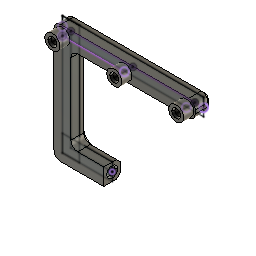
ThymioPipeRight (Autodesk Fusion 360 design; units mm, degrees)
part number: 2026-07-25-12-46-37-423
Autodesk Fusion 360 part; units mm, degrees
sketch "Sketch1" plane through (0, 0, 0) normal (0, 1, 0) x (1, 0, 0)
  line L0 (0, 0) -> (-20, 0)
  line L1 (-20, 0) -> (-20, -49)
  line L2 (-20, -49) -> (10, -49)
  line L3 (10, -49) -> (40, -49)
  line L4 (0, -4.1) -> (-24.1, -4.1)
  line L5 (-24.1, -4.1) -> (-24.1, 4.1)
  line L6 (-24.1, 4.1) -> (0, 4.1)
  line L7 (0, 4.1) -> (0, -4.1)
  line L8 (-24.1, 4.1) -> (-15.9, 4.1)
  line L9 (-15.9, 4.1) -> (-15.9, -53.4)
  line L10 (-15.9, -53.4) -> (-24.1, -53.4)
  line L11 (-24.1, -53.4) -> (-24.1, 4.1)
  line L12 (-24.1, -53.4) -> (44.3, -53.4)
  line L13 (44.3, -53.4) -> (44.3, -45.2)
  line L14 (44.3, -45.2) -> (-24.1, -45.2)
  line L15 (-24.1, -45.2) -> (-24.1, -53.4)
  dimension "d10" = 20
  dimension "d11" = 49
  dimension "d12" = 30
  dimension "d13" = 30
  dimension "d14" = 8.2
  dimension "d15" = 24.1
  dimension "d16" = 57.5
  dimension "d18" = 68.4
  dimension "d19" = 8.2
  dimension "d20" = 8.2
  constraint coincident L0.start origin
  constraint horizontal L0
  constraint vertical L1
  constraint horizontal L3
  constraint horizontal L2
  constraint horizontal L4
  constraint vertical L5
  constraint horizontal L6
  constraint vertical L7
  constraint midpoint L0.start L7
  constraint horizontal L8
  constraint vertical L9
  constraint horizontal L10
  constraint vertical L11
  constraint horizontal L12
  constraint vertical L13
  constraint horizontal L14
  constraint vertical L15
  measures "d10" distance of L0.start L0.end
  measures "d11" distance of L0.end L1.end
  measures "d12" distance of L1.end L2.end
  measures "d13" distance of L2.end L3.end
  measures "d14" distance of L4.start L6.end
  measures "d15" distance of L5 L7
  measures "d16" distance of L6 L10
  measures "d18" distance of L13 L15
  measures "d19" distance of L12 L14
  measures "d20" distance of L9 L11
extrude "Extrude1" add sketch "Sketch1" along normal mid plane 8.2
sketch "Sketch2" plane through (0, -4.1, 0) normal (0, -1, 0) x (1, 0, 0)
  line L0 (-24.1, 53.4) -> (-24.1, -4.1)
  line L1 (-24.1, -4.1) -> (0, -4.1)
  line L2 (0, -4.1) -> (0, 4.1)
  line L3 (0, 4.1) -> (-15.9, 4.1)
  line L4 (-15.9, 4.1) -> (-15.9, 45.2)
  line L5 (-15.9, 45.2) -> (44.3, 45.2)
  line L6 (44.3, 45.2) -> (44.3, 53.4)
  line L7 (44.3, 53.4) -> (-24.1, 53.4)
  line L8 (-20, 49) -> (10, 49)
  line L9 (10, 49) -> (40, 49)
  circle A0 centre (-20, 49) radius 3.625
  circle A1 centre (10, 49) radius 3.625
  circle A2 centre (40, 49) radius 3.625
  point P0 (10, 49)
  point P1 (40, 49)
  dimension "d23" = 7.25
  dimension "d24" = 7.25
  dimension "d25" = 7.25
  constraint coincident L8.start A0.centre
  constraint coincident P0 L8.end
  constraint coincident P1 L9.end
  measures "d23" diameter of A0
  measures "d24" diameter of A1
  measures "d25" diameter of A2
ref_plane "WorkPlane1" through (0, 0, 49) normal (0, 0, 1) x (1, 0, 0)
sketch "Sketch3" plane through (0, 0, 49) normal (0, 0, 1) x (1, 0, 0)
  line L0 (40, 0) -> (40, -9)
  line L1 (10, 0) -> (10, -9)
  line L2 (-20, 0) -> (-20, -9)
  line L3 (-24.1, 0) -> (44.3, 0)
  line L4 (-20, -4.1) -> (10, -4.1)
  point P0 (-20, -4.1)
  point P1 (10, -4.1)
  point P2 (40, -4.1)
  point P3 (-20, 0)
  point P4 (10, 0)
  point P5 (40, 0)
  dimension "d31" = 9
  dimension "d32" = 9
  dimension "d33" = 9
  constraint vertical L0
  constraint vertical L1
  constraint vertical L2
  constraint coincident L2 P0
  constraint coincident P5 L3
  constraint coincident P3 L2.start
  constraint coincident L1.start P4
  constraint coincident P5 L0.start
  measures "d31" distance of P5 L0.end
  measures "d32" distance of L1.end L1.start
  measures "d33" distance of L2.end P3
extrude "Extrude2" add sketch "Sketch2" along normal blind 4.9 contours L8 L9 A1 | L8 L9 A1 | A0 | A2
pipe "Pipe1" cut diameter 4.2 path "Sketch1" along L0 L1 L2 L3
pipe "Pipe2" cut diameter 3.25 path "Sketch3" along L2
pipe "Pipe3" cut diameter 3.25 path "Sketch3" along L1
pipe "Pipe4" cut diameter 3.25 path "Sketch3" along L0
fillet "Fillet1" offset 0.5 second offset 1 3 edges at (8.485, -9, 49.5876) (-21.515, -9, 49.5876) (38.485, -9, 49.5876) measured on face at (12.9388, -9, 49.2608) measured on face at (-17.0567, -9, 48.7794) measured on face at (42.9433, -9, 49.2206)
fillet "Fillet1" offset 0.5 second offset 1 1 edges at (0, 1.9579, -0.7594) measured on face at (0, 3.4314, 0.0523)
fillet "Fillet2" radius 3.25 6 edges at (-15.9, 0, 45.2) (44.3, 0, 45.2) (44.3, 0, 53.4) (-24.1, 0, 53.4) (-24.1, 0, -4.1) (-15.9, 0, 4.1)
sketch "Sketch4" plane through (0, 4.1, 0) normal (0, 1, 0) x (1, 0, 0)
  line L0 (-12.0349, 3.5252) -> (-22.5468, 3.5252) construction
  line L1 (-22.5468, 3.5252) -> (-22.5468, -4.1335) construction
  line L2 (-22.5468, -4.1335) -> (-12.0349, -4.1335) construction
  line L3 (-12.0349, -4.1335) -> (-12.0349, 3.5252) construction
  arc A0 (-21.1, 4.1) -> (-24.1, 1.1) centre (-21.1, 1.1) ccw
  line L4 (-24.1, 1.1) -> (-24.1, -50.4)
  arc A1 (-24.1, -50.4) -> (-21.1, -53.4) centre (-21.1, -50.4) ccw
  line L5 (-21.1, -53.4) -> (41.3, -53.4)
  arc A2 (41.3, -53.4) -> (44.3, -50.4) centre (41.3, -50.4) ccw
  line L6 (44.3, -50.4) -> (44.3, -48.2)
  arc A3 (44.3, -48.2) -> (41.3, -45.2) centre (41.3, -48.2) ccw
  line L7 (41.3, -45.2) -> (-12.9, -45.2)
  arc A4 (-15.9, -42.2) -> (-12.9, -45.2) centre (-12.9, -42.2) ccw
  line L8 (-15.9, -42.2) -> (-15.9, -7.1)
  arc A5 (-12.9, -4.1) -> (-15.9, -7.1) centre (-12.9, -7.1) ccw
  line L9 (-12.9, -4.1) -> (0, -4.1)
  line L10 (0, -4.1) -> (0, 4.1)
  line L11 (0, 4.1) -> (-21.1, 4.1)
  dimension "d60" = 6
  dimension "d61" = 0
extrude "Extrude3" [suppressed]
extrude "Extrude4" [suppressed]
chamfer "Chamfer1" distance 2 angle 45 13 edges at (-24.1, 4.1, 24.65) (-23.1481, 4.1, 52.4481) (10.1, 4.1, 53.4) (43.3481, 4.1, 52.4481) (44.3, 4.1, 49.3) (43.3481, 4.1, 46.1519) (14.2, 4.1, 45.2) (-14.9481, 4.1, 44.2481) (-15.9, 4.1, 24.65) (-14.9481, 4.1, 5.0519) (-6.325, 4.1, 4.1) (-10.425, 4.1, -4.1) (-23.1481, 4.1, -3.1481) tangent chain off
equation "WallThickness = 2 mm"
equation "SizeA = 20 mm"
equation "SizeB = 49 mm"
equation "SizeC = 30 mm"
equation "SizeD = 30 mm"
equation "SizeK = 7 mm + 2 mm"
equation "PumpHoleDiameter = 4.2 mm"
equation "ValveHoleDiameter = 3.25 mm"
equation "d10 = SizeA"
equation "d11 = SizeB"
equation "d12 = SizeC"
equation "d13 = SizeD"
equation "d14 = WallThickness * 2 + PumpHoleDiameter"
equation "d15 = SizeA + WallThickness + PumpHoleDiameter / 2"
equation "d16 = SizeB + 2 * PumpHoleDiameter - 2 * WallThickness + PumpHoleDiameter * 1 / 2 + WallThickness"
equation "d18 = SizeC + SizeD + 2 * PumpHoleDiameter"
equation "d19 = PumpHoleDiameter * 1 + WallThickness * 2"
equation "d20 = PumpHoleDiameter + 2 * WallThickness"
equation "d21 = PumpHoleDiameter / 2 + WallThickness"
equation "d23 = ValveHoleDiameter + 2 * WallThickness"
equation "d24 = ValveHoleDiameter + 2 * WallThickness"
equation "d25 = ValveHoleDiameter + 2 * WallThickness"
equation "d29 = SizeB"
equation "d31 = SizeK"
equation "d32 = SizeK"
equation "d33 = SizeK"
equation "d34 = SizeK - ( PumpHoleDiameter / 2 + WallThickness )"
equation "d38 = PumpHoleDiameter"
equation "d42 = ValveHoleDiameter"
equation "d46 = ValveHoleDiameter"
equation "d50 = ValveHoleDiameter"
equation "d59 = min(ValveHoleDiameter; PumpHoleDiameter)"
equation "d61 = 'v2'"
